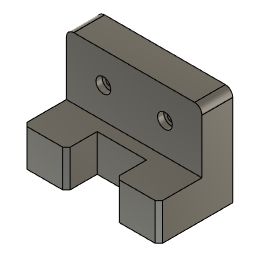
Mount_Bracket v1 (Autodesk Fusion 360 design; units mm, degrees)
Autodesk Fusion 360 part; units mm, degrees
sketch "Sketch1" plane through (0, 0, 0) normal (0, 0, 1) x (1, 0, 0)
  line L0 (0, 0) -> (110, 0)
  line L1 (110, 0) -> (110, 60)
  line L2 (110, 60) -> (0, 60)
  line L3 (0, 60) -> (0, 0)
  line L4 (0, 60) -> (110, 60)
  line L5 (110, 60) -> (110, 35)
  line L6 (110, 35) -> (0, 35)
  line L7 (0, 35) -> (0, 60)
  line L8 (75, 25) -> (35, 25)
  line L9 (35, 25) -> (35, 0)
  line L10 (75, 0) -> (75, 25)
  line L11 (75, 25) -> (35, -25) construction
  line L12 (35, 25) -> (75, -25) construction
  point P0 (55, 0)
  dimension "d12" = 110
  dimension "d13" = 60
  dimension "d14" = 110
  dimension "d15" = 25
  dimension "d16" = 40
  dimension "d17" = 50
  constraint horizontal L0
  constraint vertical L1
  constraint horizontal L2
  constraint vertical L3
  constraint coincident L0.start L3.end
  constraint horizontal L4
  constraint vertical L5
  constraint horizontal L6
  constraint vertical L7
  constraint horizontal L8
  constraint perpendicular L8 L9
  constraint parallel L9 L10
  constraint coincident L11 P0
  constraint coincident L12 P0
  constraint midpoint L0 P0
  constraint coincident L0 L10.start
  constraint coincident L0 L9.end
  measures "d12" distance of L0.start L0.end
  measures "d13" distance of L0.start L2.end
  measures "d14" distance of L2.end L1.end
  measures "d15" distance of L2.end L6.end
  measures "d16" distance of L11.end L12.end
  measures "d17" distance of L8.end L11.end
extrude "Extrude1" add sketch "Sketch1" along normal blind 30 contours L0 L1 L3 L6 L8 L9 L10
extrude "Extrude2" add sketch "Sketch1" along normal blind 80 contours L1 L2 L3 L4 L5 L6 L7
fillet "Fillet1" radius 6 2 edges at (110, 47.5, 80) (0, 47.5, 80)
chamfer "Chamfer1" distance 3 angle 45 4 edges at (110, 0, 15) (75, 0, 15) (35, 0, 15) (0, 0, 15)
sketch "Sketch2" plane through (0, 35, 0) normal (0, -1, 0) x (1, 0, 0)
  arc A0 (6, 80) -> (0, 74) centre (6, 74) ccw
  line L0 (0, 74) -> (0, 30)
  line L1 (0, 30) -> (110, 30)
  line L2 (110, 30) -> (110, 74)
  arc A1 (110, 74) -> (104, 80) centre (104, 74) ccw
  line L3 (104, 80) -> (6, 80)
  line L4 (55, 80) -> (55, 30) construction
  circle A2 centre (80, 55) radius 6
  circle A3 centre (80, 55) radius 3
  circle A4 centre (30, 55) radius 6
  circle A5 centre (30, 55) radius 3
  dimension "d27" = 12
  dimension "d28" = 6
  dimension "d29" = 25
  dimension "d32" = 25
  constraint midpoint L3 L4.start
  constraint midpoint L1 L4.end
  constraint concentric A2 A3
  constraint symmetric L4 A2 A4
  constraint symmetric L4 A3 A5
  measures "d27" diameter of A2
  measures "d28" diameter of A3
  measures "d29" distance of L3 A2.centre
  measures "d32" distance of L4 A2.centre
extrude "Extrude3" cut sketch "Sketch2" against normal blind 25 contours A3 | A5
extrude "Extrude4" cut sketch "Sketch2" against normal blind 5 contours A4
extrude "Extrude5" cut sketch "Sketch2" against normal blind 5 contours A2
equation "width = 60 mm"
equation "length = 110 mm"
equation "base_height = 30 mm"
equation "back_height = 80 mm"
equation "back_width = 25 mm"
equation "countersink_diameter = 12 mm"
equation "hole_diameter = 6 mm"
equation "countersink_depth = 5 mm"
equation "cut_depth = 25 mm"
equation "cut_width = 40 mm"
equation "d12 = length"
equation "d13 = width"
equation "d14 = length"
equation "d15 = back_width"
equation "d16 = cut_width"
equation "d17 = cut_depth * 2"
equation "top_radius = 6 mm"
equation "d19 = base_height"
equation "d21 = back_height"
equation "d24 = top_radius"
equation "chamfer = 3 mm"
equation "d26 = chamfer"
equation "d27 = countersink_diameter"
equation "d28 = hole_diameter"
equation "d29 = hole_distance_from_top"
equation "hole_distance_from_top = 25 mm"
equation "distance_between_holes = 50 mm"
equation "d32 = distance_between_holes / 2"
equation "d33 = -back_width"
equation "d35 = -countersink_depth"
equation "d37 = -countersink_depth"
